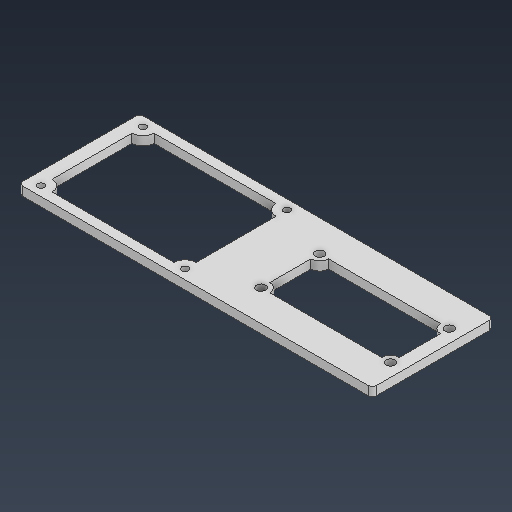
# Autodesk Inventor part: motherboard
Saved by Autodesk Inventor 2026.1 (Build 301233020, 233B)
## iProperties
Created: 2025-12-15
Part Number: motherboard
Material: Generic
Document SubType Name: Modeling
Designer: Piter
Density: 1 g/cm^3
Appearance: Default
Author: Piter
Autodesk Inventor part; units mm, degrees
ref_plane "YZ Plane" through (0, 0, 0) normal (1, 0, 0) x (0, 1, 0)
ref_plane "XZ Plane" through (0, 0, 0) normal (0, 1, 0) x (-1, 0, 0)
ref_plane "XY Plane" through (0, 0, 0) normal (0, 0, 1) x (1, 0, 0)
sketch "Sketch1" plane through (0, 0, 0) normal (0, 1, 0) x (-1, 0, 0)
  line L0 (-80, 27.5) -> (80, 27.5)
  line L1 (80, 27.5) -> (80, -27.5)
  line L2 (80, -27.5) -> (-80, -27.5)
  line L3 (-80, -27.5) -> (-80, 27.5)
  line L4 (-80, 27.5) -> (80, -27.5) construction
  line L5 (80, 27.5) -> (-80, -27.5) construction
  point P0 (0, 0)
  dimension "d0" = 160
  dimension "d1" = 55
  constraints: 12 end point, 2 midpoint, 2 parallel, 1 horizontal, 1 perpendicular
  measures "d0" distance of L1.end L2.end
  measures "d1" distance of L0.end L1.end
extrude "Extrusion1" add sketch "Sketch1" along normal blind 4
sketch "Sketch2" plane through (0, 4, 0) normal (0, 1, 0) x (1, 0, 0)
  line L0 (80, 27.5) -> (-80, 27.5) projected
  line L1 (-80, 27.5) -> (-80, -27.5) projected
  line L2 (-80, -27.5) -> (80, -27.5) projected
  line L3 (80, -27.5) -> (80, 27.5) projected
  line L4 (-74, -23) -> (-9, -23)
  line L5 (-9, -23) -> (-9, 23)
  line L6 (-9, 23) -> (-74, 23)
  line L7 (-74, 23) -> (-74, -23)
  line L8 (-74, -23) -> (-74, -27.5)
  line L9 (-74, 23) -> (-74, 27.5)
  circle A0 centre (-74, -23) radius 1.55
  circle A1 centre (-74, 23) radius 1.55
  circle A2 centre (-9, -23) radius 1.55
  circle A3 centre (-9, 23) radius 1.55
  circle A4 centre (-74, 23) radius 5
  circle A5 centre (-9, 23) radius 5
  circle A6 centre (-74, -23) radius 5
  circle A7 centre (-9, -23) radius 5
  line L10 (-80, 0) -> (80, 0) construction
  line L11 (15.5, -13.25) -> (74, -13.25)
  line L12 (74, -13.25) -> (74, 13.25)
  line L13 (74, 13.25) -> (15.5, 13.25)
  line L14 (15.5, 13.25) -> (15.5, -13.25)
  line L15 (15.5, -13.25) -> (74, 13.25) construction
  line L16 (74, -13.25) -> (15.5, 13.25) construction
  circle A8 centre (15.5, -13.25) radius 2.05
  circle A9 centre (15.5, 13.25) radius 2.05
  circle A10 centre (74, 13.25) radius 2.05
  circle A11 centre (74, -13.25) radius 2.05
  circle A12 centre (15.5, 13.25) radius 4
  circle A13 centre (15.5, -13.25) radius 4
  circle A14 centre (74, -13.25) radius 4
  circle A15 centre (74, 13.25) radius 4
  point P0 (0, 0)
  point P1 (44.75, 0)
  point P2 (74, 9.25)
  point P3 (70, 13.25)
  point P4 (19.5, 13.25)
  point P5 (15.5, 9.25)
  point P6 (15.5, -9.25)
  point P7 (19.5, -13.25)
  point P8 (70, -13.25)
  point P9 (74, -9.25)
  point P10 (-14, -23)
  point P11 (-9, -18)
  point P12 (-9, 18)
  point P13 (-14, 23)
  point P14 (-69, 23)
  point P15 (-74, 18)
  point P16 (-74, -18)
  point P17 (-69, -23)
  dimension "d4" = 65
  dimension "d5" = 46
  dimension "d6" = 3.1
  dimension "d7" = 3.1
  dimension "d8" = 3.1
  dimension "d9" = 3.1
  dimension "d10" = 6
  dimension "d11" = 10
  dimension "d12" = 10
  dimension "d13" = 10
  dimension "d14" = 10
  dimension "d15" = 58.5
  dimension "d16" = 26.5
  dimension "d17" = 6
  dimension "d18" = 4.1
  dimension "d19" = 4.1
  dimension "d20" = 4.1
  dimension "d21" = 4.1
  dimension "d22" = 8
  dimension "d23" = 8
  dimension "d24" = 8
  dimension "d25" = 8
  constraints: 26 end point, 16 centre point, 16 coincident, 4 midpoint, 4 parallel, 4 point on line, 2 horizontal, 2 perpendicular, 1 collinear, 1 vertical
  measures "d4" distance of L6.end L5.end
  measures "d5" distance of L5.end L4.end
  measures "d6" diameter of A0
  measures "d7" diameter of A1
  measures "d8" diameter of A2
  measures "d9" diameter of A3
  measures "d10" distance from line of L1 A1.centre
  measures "d11" diameter of A4
  measures "d12" diameter of A5
  measures "d13" diameter of A6
  measures "d14" diameter of A7
  measures "d15" distance of L13.end L12.end
  measures "d16" distance of L12.end L11.end
  measures "d17" distance between parallel lines of L3 L12
  measures "d18" diameter of A8
  measures "d19" diameter of A9
  measures "d20" diameter of A10
  measures "d21" diameter of A11
  measures "d22" diameter of A12
  measures "d23" diameter of A13
  measures "d24" diameter of A14
  measures "d25" diameter of A15
extrude "Extrusion2" cut sketch "Sketch2" against normal blind 10 contours A5 L5 A7 L4 A6 L7 A4 L6 | A3 L5 L6 | L6 L5 A3 | A1 L6 L9 | L9 L7 A1 | A1 L7 L6 | A2 L4 L5 | L5 L4 A2 | A0 L7 L8 | L8 L4 A0 | L4 L7 A0 | L14 A8 L11 | L11 A8 L14 | A13 L14 A12 L13 A15 L12 A14 L11 | A11 L12 L11 | L11 L12 A11 | A9 L13 L14 | L14 L13 A9 | A10 L13 L12 | L12 L13 A10
fillet "Fillet1" radius 2 4 edges at (-80, 2, 27.5) (80, 2, 27.5) (80, 2, -27.5) (-80, 2, -27.5)
sketch "Sketch3" plane through (0, 0, 0) normal (0, -1, 0) x (1, 0, 0)
  circle A0 centre (-9, 23) radius 1.55 projected
  circle A1 centre (15.5, -13.25) radius 2.05 projected
  circle A2 centre (-74, -23) radius 1.55 projected
  circle A3 centre (74, -13.25) radius 2.05 projected
  arc A4 (19.5, -13.25) -> (15.5, -9.25) centre (15.5, -13.25) ccw projected
  line L0 (15.5, -9.25) -> (15.5, 9.25) projected
  arc A5 (15.5, 9.25) -> (19.5, 13.25) centre (15.5, 13.25) ccw projected
  line L1 (19.5, 13.25) -> (70, 13.25) projected
  arc A6 (70, 13.25) -> (74, 9.25) centre (74, 13.25) ccw projected
  line L2 (74, 9.25) -> (74, -9.25) projected
  arc A7 (74, -9.25) -> (70, -13.25) centre (74, -13.25) ccw projected
  line L3 (70, -13.25) -> (19.5, -13.25) projected
  circle A8 centre (15.5, 13.25) radius 2.05 projected
  circle A9 centre (-9, -23) radius 1.55 projected
  circle A10 centre (-74, 23) radius 1.55 projected
  circle A11 centre (74, 13.25) radius 2.05 projected
  arc A12 (-9, -18) -> (-14, -23) centre (-9, -23) ccw projected
  line L4 (-14, -23) -> (-69, -23) projected
  arc A13 (-69, -23) -> (-74, -18) centre (-74, -23) ccw projected
  line L5 (-74, -18) -> (-74, 18) projected
  arc A14 (-74, 18) -> (-69, 23) centre (-74, 23) ccw projected
  line L6 (-69, 23) -> (-14, 23) projected
  arc A15 (-14, 23) -> (-9, 18) centre (-9, 23) ccw projected
  line L7 (-9, 18) -> (-9, -18) projected
  arc A16 (-80, -25.5) -> (-78, -27.5) centre (-78, -25.5) ccw projected
  line L8 (78, -27.5) -> (-78, -27.5) projected
  arc A17 (78, -27.5) -> (80, -25.5) centre (78, -25.5) ccw projected
  line L9 (80, 25.5) -> (80, -25.5) projected
  arc A18 (80, 25.5) -> (78, 27.5) centre (78, 25.5) ccw projected
  line L10 (-78, 27.5) -> (78, 27.5) projected
  arc A19 (-78, 27.5) -> (-80, 25.5) centre (-78, 25.5) ccw projected
  line L11 (-80, -25.5) -> (-80, 25.5) projected
  arc A20 (79.8, 25.5) -> (78, 27.3) centre (78, 25.5) ccw
  line L12 (79.8, 25.5) -> (79.8, -25.5)
  arc A21 (78, -27.3) -> (79.8, -25.5) centre (78, -25.5) ccw
  line L13 (78, -27.3) -> (-78, -27.3)
  arc A22 (-79.8, -25.5) -> (-78, -27.3) centre (-78, -25.5) ccw
  line L14 (-79.8, -25.5) -> (-79.8, 25.5)
  arc A23 (-78, 27.3) -> (-79.8, 25.5) centre (-78, 25.5) ccw
  line L15 (-78, 27.3) -> (78, 27.3)
  point P0 (0, 0)
  dimension "d29" = 0.2
  constraints: 8 end point, 8 point on circle, 4 centre point, 7 other
  measures "d29" distance between parallel lines of L10 L15
extrude "offset" cut sketch "Sketch3" against normal through all contours L11 A19 L10 A18 L9 A17 L8 A16
body "Solid1"
